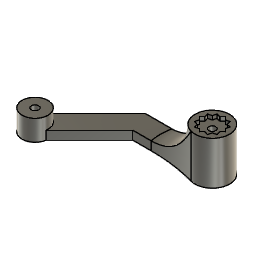
wheel_aligment_arm_right_20mm_offset (Autodesk Fusion 360 design; units mm, degrees)
Autodesk Fusion 360 part; units mm, degrees
sketch "Sketch1" plane through (0, 0, 0) normal (0, 0, 1) x (1, 0, 0)
  line L0 (0, 0) -> (40, 0)
  line L1 (40, 12) -> (0, 12)
  line L2 (0, 12) -> (0, 0)
  line L3 (40, 0) -> (68.2843, -28.2843)
  line L4 (40, 0) -> (80, 0) construction
  line L5 (68.2843, -28.2843) -> (76.7696, -19.799)
  line L6 (76.7696, -19.799) -> (44.9706, 12)
  line L7 (40, 12) -> (44.9706, 12)
  circle A0 centre (0, 6) radius 10
  line L8 (0, 6) -> (0, 13.5) construction
  line L9 (0, 13.5) -> (0, -1.5) construction
  line L10 (0, 6) -> (7.5, 6) construction
  line L11 (7.5, 6) -> (-7.5, 6) construction
  line L12 (-7.5, 6) -> (0, 13.5)
  line L13 (0, 13.5) -> (7.5, 6)
  line L14 (7.5, 6) -> (0, -1.5)
  line L15 (0, -1.5) -> (-7.5, 6)
  line L16 (0, 6) -> (3.75, 12.4952) construction
  line L17 (3.75, 12.4952) -> (-3.75, -0.4952) construction
  line L18 (0, 6) -> (6.4952, 2.25) construction
  line L19 (6.4952, 2.25) -> (-6.4952, 9.75) construction
  line L20 (-6.4952, 9.75) -> (3.75, 12.4952)
  line L21 (3.75, 12.4952) -> (6.4952, 2.25)
  line L22 (6.4952, 2.25) -> (-3.75, -0.4952)
  line L23 (-3.75, -0.4952) -> (-6.4952, 9.75)
  line L24 (0, 6) -> (6.4952, 9.75) construction
  line L25 (0, 6) -> (7.5, 6) construction
  line L26 (6.4952, 9.75) -> (-6.4952, 2.25) construction
  line L27 (0, 6) -> (3.75, -0.4952) construction
  line L28 (3.75, -0.4952) -> (-3.75, 12.4952) construction
  line L29 (-3.75, 12.4952) -> (-6.4952, 2.25)
  line L30 (-6.4952, 2.25) -> (3.75, -0.4952)
  line L31 (3.75, -0.4952) -> (6.4952, 9.75)
  line L32 (6.4952, 9.75) -> (-3.75, 12.4952)
  circle A1 centre (0, 6) radius 2
  circle A2 centre (72.5269, -24.0416) radius 7.5
  line L33 (76.1769, -26.149) -> (76.1769, -21.9343)
  line L34 (76.1769, -21.9343) -> (72.5269, -19.827)
  line L35 (72.5269, -19.827) -> (68.8769, -21.9343)
  line L36 (68.8769, -21.9343) -> (68.8769, -26.149)
  line L37 (68.8769, -26.149) -> (72.5269, -28.2563)
  line L38 (72.5269, -28.2563) -> (76.1769, -26.149)
  line L39 (68.8769, -21.9343) -> (68.8769, -17.4897)
  line L40 (76.1769, -21.9343) -> (76.1769, -17.4897)
  circle A3 centre (72.5269, -24.0416) radius 2.1
  point P0 (72.5269, -24.0416)
  dimension "d1" = 40
  dimension "d2" = 12
  dimension "d3" = 40
  dimension "d4" = 45
  dimension "d5" = 12
  dimension "d8" = 7.5
  dimension "d9" = 15
  dimension "d10" = 7.5
  dimension "d11" = 15
  dimension "d12" = 7.5
  dimension "d13" = 30
  dimension "d14" = 15
  dimension "d15" = 7.5
  dimension "d16" = 90
  dimension "d17" = 15
  dimension "d18" = 30
  dimension "d19" = 7.5
  dimension "d20" = 15
  dimension "d21" = 7.5
  dimension "d22" = 15
  dimension "d23" = 20
  dimension "d24" = 4
  dimension "d25" = 15
  dimension "d35" = 3.65
  dimension "d39" = 4.2
  dimension "d42" = 180
  constraint horizontal L0
  constraint horizontal L1
  constraint vertical L2
  constraint coincident L0.start L2.end
  constraint horizontal L4
  constraint perpendicular L3 L5
  constraint perpendicular L5 L6
  constraint midpoint L2 A0.centre
  constraint coincident A0.centre L8.start
  constraint parallel L2 L8
  constraint perpendicular L0 L9
  constraint perpendicular L8 L10
  constraint parallel L10 L11
  constraint parallel L16 L17
  constraint perpendicular L16 L19
  constraint horizontal L25
  constraint parallel L24 L26
  constraint perpendicular L24 L27
  constraint parallel L27 L28
  constraint midpoint L5 P0
  constraint coincident P0 A2.centre
  constraint vertical L39
  constraint coincident A2 L39.end
  constraint vertical L40
  constraint coincident A2 L40.end
  measures "d1" distance of L0.start L0.end
  measures "d2" distance of L0.start L1.end
  measures "d3" distance of L0.end L3.end
  measures "d4" angle of L3 L4
  measures "d5" distance of L3.end L5.end
  measures "d8" distance of A0.centre L8.end
  measures "d9" distance of L8.end L9.end
  measures "d10" distance of A0.centre L10.end
  measures "d11" distance of L10.end L11.end
  measures "d12" distance of A0.centre L16.end
  measures "d13" angle of L9 L16
  measures "d14" distance of L16.end L17.end
  measures "d15" distance of A0.centre L18.end
  measures "d16" angle of L17 L18
  measures "d17" distance of L18.end L19.end
  measures "d18" angle of L24 L25
  measures "d19" distance of A0.centre L24.end
  measures "d20" distance of L24.end L26.end
  measures "d21" distance of A0.centre L27.end
  measures "d22" distance of L27.end L28.end
  measures "d23" diameter of A0
  measures "d24" diameter of A1
  measures "d25" diameter of A2
  measures "d35" distance of P0 L38
  measures "d39" diameter of A3
  measures "d42" angle of L36 L39 L0.start
extrude "Extrude1" add sketch "Sketch1" against normal blind 5
extrude "Extrude9" add sketch "Sketch1" against normal blind 25 contours L0 L2 L14 L30 | L0 L2 L14 L15 L22 | L0 L14 L30 | L0 L1 A0 L12 L13 L14 L15 L20 L21 L22 L23 L29 L30 L31 L32 | L2 L12 L15 L20 L23 L29 L30 A1 | L2 L13 L14 L21 L22 L31 L32 A1 | L15 L22 L30 | L14 L22 L30 | L0 L14 L22 L30 L31 | L0 L30 L31 | L2 A1 | L2 A1 | L14 L22 L31 | L15 L22 L23 L30 | L15 L23 L30 | L0 L1 A0 L13 L14 L21 L22 L31 L32 | L14 L21 L31 | L14 L21 L22 L31 | L15 L23 L29 L30 | L15 L23 L29 | L1 L2 L12 L13 L32 | L1 L2 L13 L20 | L13 L20 L32 | L12 L20 L32 | L13 L14 L21 L31 | L13 L21 L31 | L12 L15 L23 L29 | L12 L23 L29 | L12 L20 L29 L32 | L12 L20 L29 | L1 L13 L20 L21 L32 | L1 L13 L20 | L13 L21 L32 | L13 L21 L31 L32 | L12 L20 L23 L29 | L1 L20 L21
extrude "Extrude2" cut sketch "Sketch1" along normal blind 2.2 from surface at -25 contours L0 L2 L14 L30 | L0 L2 L14 L15 L22 | L0 L14 L30 | L2 L12 L15 L20 L23 L29 L30 A1 | L2 L13 L14 L21 L22 L31 L32 A1 | L15 L22 L30 | L14 L22 L30 | L0 L14 L22 L30 L31 | L0 L30 L31 | L2 A1 | L2 A1 | L14 L22 L31 | L15 L22 L23 L30 | L15 L23 L30 | L14 L21 L31 | L14 L21 L22 L31 | L15 L23 L29 L30 | L15 L23 L29 | L1 L2 L12 L13 L32 | L1 L2 L13 L20 | L13 L20 L32 | L12 L20 L32 | L13 L14 L21 L31 | L13 L21 L31 | L12 L15 L23 L29 | L12 L23 L29 | L12 L20 L29 L32 | L12 L20 L29 | L1 L13 L20 L21 L32 | L1 L13 L20 | L13 L21 L32 | L13 L21 L31 L32 | L12 L20 L23 L29 | L1 L20 L21
extrude "Extrude3" cut sketch "Sketch1" against normal blind 25 contours L2 A1 | L2 A1
extrude "Extrude4" add sketch "Sketch1" against normal blind 12 contours L3 L5 A2 L36 L37 L39 | L3 L5 L6 A2 L33 L37 L38 L40 | L5 L6 A2 L34 L35 L39 L40 | L5 L34 L35 L36 L37 A3 | L5 L33 L34 L37 L38 A3 | L6 A2 L40 | L5 A3 | L5 A3 | L5 L6 L40 | L5 L34 L40
extrude "Extrude5" cut sketch "Sketch1" along normal mid plane 4 from surface at -7 contours L5 L6 A2 L34 L35 L39 L40 | L5 L34 L35 L36 L37 A3 | L5 L33 L34 L37 L38 A3 | L6 A2 L40 | L5 A3 | L5 A3 | L5 L34 L40
extrude "Extrude6" cut sketch "Sketch1" against normal blind 12 contours L5 A3 | L5 A3
move_body "Move1" bodies 1 to x (-1, 0, 0) y (0, 1, 0) z (0, 0, -1) at (-20, 0, -50)
move_body "Move2" bodies 1 to x (1, 0, 0) y (0, 1, 0) z (0, 0, 1) at (20, 0, 50)
move_body "Move3" bodies 1 to x (1, 0, 0) y (0, 1, 0) z (0, 0, 1) at (-0.21, 0.1034, 0.1851)
fillet "Fillet1" radius 20 1 edges at (-10.21, 6.1034, 5.1851)
fillet "Fillet2" radius 100 2 edges at (-8.21, 0.1034, 12.6851) (-8.21, 12.1034, 12.6851)
equation "d13 = ( 90 / 3 ) * 1 deg"
